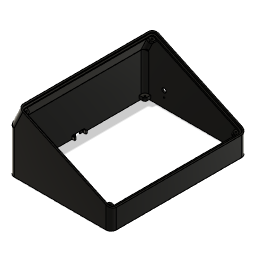
CP-BO Side v19 (Autodesk Fusion 360 design; units mm, degrees)
Autodesk Fusion 360 part; units mm, degrees
sketch "Esquisse1" plane through (0, 0, 0) normal (0, 0, 1) x (1, 0, 0)
  line L0 (17.7197, 122.5237) -> (198.9812, 38)
  line L1 (198.9812, 38) -> (0, 38) construction
  line L2 (198.9812, 38) -> (179.1229, -4.5863) construction
  line L3 (181.2616, 0) -> (-66.8807, 115.7106) construction
  line L4 (17.7197, 122.5237) -> (0, 84.5237)
  line L5 (0, 84.5237) -> (0, 0)
  line L6 (198.9812, 38) -> (198.9812, 0)
  line L7 (2.6, 0) -> (2.6, 83.3113) construction
  line L8 (0, 0) -> (198.9812, 0)
  line L9 (80, 0) -> (80, 93.4819) construction
  line L10 (20.0761, 121.4248) -> (0, 78.3715) construction
  dimension "d7" = 25
  dimension "d8" = 200
  dimension "d13" = 46.188
  dimension "d15" = 2.6
  dimension "d17" = 38
  dimension "d20" = 83.1247
  dimension "d21" = 197.5823
  dimension "d188" = 80
  dimension "d189" = 2.6
  dimension "d190" = 41.9284
  constraint perpendicular L0 L2
  constraint coincident L2 L3.start
  constraint parallel L0 L3
  constraint coincident L3 L4.end
  constraint perpendicular L3 L4
  constraint perpendicular L1 L6
  constraint coincident L3 L7.end
  constraint perpendicular L6 L8
  constraint coincident L3.start L8
  constraint perpendicular L5 L8
  constraint coincident L5.end L8.start
  constraint coincident L7.start L8
  constraint coincident L8 L9.start
  constraint perpendicular L8 L9
  constraint coincident L1.end L5
  constraint coincident L0 L9.end
  constraint vertical L9
  constraint coincident L0 L10.start
  constraint coincident L5 L10.end
  constraint parallel L4 L10
  measures "d7" angle of L0 L1
  measures "d8" distance of L0.start L0.end
  measures "d15" distance of L5 L7
  measures "d17" distance of L6.end L0.end
  measures "d188" distance of L5 L9
  measures "d189" distance of L4 L10
  measures "d190" distance of L3 L10.start
extrude "Largeur boitier" add sketch "Esquisse1" along normal blind 265 makes body 1
fillet "Congés boitier" radius 10 6 edges at (198.9812, 19, 0) (198.9812, 19, 265) (0, 42.2618, 265) (8.8598, 103.5237, 265) (8.8598, 103.5237, 0) (0, 42.2618, 0) on bodies 1
fillet "Congé arrière" radius 10 3 edges at (2.9289, 83.8743, 2.9289) (0, 84.5237, 132.5) (2.9289, 83.8743, 262.0711) on bodies 1
sketch "Esquisse6" plane through (50.0941, 107.4272, 0) normal (0.422618, 0.906308, 0) x (0, 0, -1)
  arc A0 (0, 25.7212) -> (-10, 35.7212) centre (-10, 25.7212) ccw
  line L0 (-10, 35.7212) -> (-255, 35.7212)
  arc A1 (-255, 35.7212) -> (-265, 25.7212) centre (-255, 25.7212) ccw
  line L1 (-265, 25.7212) -> (-265, -153.245)
  ellipse E0 centre (-255, -153.245) end of major axis (-255, -164.2788) minor radius 10 (-265, -153.245) -> (-255, -164.2788) ccw
  line L2 (-255, -164.2788) -> (-10, -164.2788)
  ellipse E1 centre (-10, -153.245) end of major axis (-10, -164.2788) minor radius 10 (-10, -164.2788) -> (0, -153.245) ccw
  line L3 (0, -153.245) -> (0, 25.7212)
  line L4 (-262.4, 25.7212) -> (-262.4, -153.245)
  spline S0 degree 3 poles (-262.4, -153.245) (-262.4, -155.3628) (-261.6582, -157.4606) (-260.4214, -158.9788) (-259.0049, -160.7177) (-256.9935, -161.6788) (-255, -161.6788) knots -1.570796 -1.570796 -1.570796 -1.570796 -0.838623 -0.838623 -0.838623 0 0 0 0
  line L5 (-255, -161.6788) -> (-10, -161.6788)
  spline S1 degree 3 poles (-10, -161.6788) (-8.1331, -161.6788) (-6.2517, -160.8417) (-4.8554, -159.301) (-3.5538, -157.8648) (-2.7132, -155.8209) (-2.6111, -153.7066) (-2.6037, -153.5529) (-2.6, -153.3989) (-2.6, -153.245) knots 0 0 0 0 0.785398 0.785398 0.785398 1.517572 1.517572 1.517572 1.570796 1.570796 1.570796 1.570796
  line L6 (-2.6, -153.245) -> (-2.6, 25.7212)
  arc A2 (-2.6, 25.7212) -> (-10, 33.1212) centre (-10, 25.7212) ccw
  line L7 (-10, 33.1212) -> (-255, 33.1212)
  arc A3 (-255, 33.1212) -> (-262.4, 25.7212) centre (-255, 25.7212) ccw
  dimension "d61" = -2.6
extrude "Trou supérieur (1)" cut sketch "Esquisse6" against normal blind 41.928 contours L4 S0 L5 S1 L6 A2 L7 A3 bodies 1
sketch "Esquisse7" plane through (0, 0, 0) normal (0, -1, 0) x (1, 0, 0)
  arc A0 (0, 10) -> (10, 0) centre (10, 10) ccw
  line L0 (10, 0) -> (188.9812, 0)
  arc A1 (188.9812, 0) -> (198.9812, 10) centre (188.9812, 10) ccw
  line L1 (198.9812, 10) -> (198.9812, 255)
  arc A2 (198.9812, 255) -> (188.9812, 265) centre (188.9812, 255) ccw
  line L2 (188.9812, 265) -> (10, 265)
  arc A3 (10, 265) -> (0, 255) centre (10, 255) ccw
  line L3 (0, 255) -> (0, 10)
  line L4 (2.6, 255) -> (2.6, 10)
  arc A4 (2.6, 10) -> (10, 2.6) centre (10, 10) ccw
  line L5 (10, 2.6) -> (188.9812, 2.6)
  arc A5 (188.9812, 2.6) -> (196.3812, 10) centre (188.9812, 10) ccw
  line L6 (196.3812, 10) -> (196.3812, 255)
  arc A6 (196.3812, 255) -> (188.9812, 262.4) centre (188.9812, 255) ccw
  line L7 (188.9812, 262.4) -> (10, 262.4)
  arc A7 (10, 262.4) -> (2.6, 255) centre (10, 255) ccw
  dimension "d64" = -2.6
extrude "Trou inférieur (2)" cut sketch "Esquisse7" against normal blind 83.311 contours L4 A4 L5 A5 L6 A6 L7 A7 bodies 1
sketch "Esquisse8" plane through (50.0941, 107.4272, 0) normal (0.422618, 0.906308, 0) x (0, 0, -1)
  line L0 (-262.4, -153.245) -> (-262.4, 25.7212)
  arc A0 (-255, 33.1212) -> (-262.4, 25.7212) centre (-255, 25.7212) ccw
  line L1 (-255, 33.1212) -> (-10, 33.1212)
  arc A1 (-2.6, 25.7212) -> (-10, 33.1212) centre (-10, 25.7212) ccw
  line L2 (-2.6, 25.7212) -> (-2.6, -153.245)
  spline S0 degree 3 poles (-2.6, -153.245) (-2.6, -153.3989) (-2.6037, -153.5529) (-2.6111, -153.7066) (-2.7132, -155.8209) (-3.5538, -157.8648) (-4.8554, -159.301) (-6.2517, -160.8417) (-8.1331, -161.6788) (-10, -161.6788) knots -1.570796 -1.570796 -1.570796 -1.570796 -1.517572 -1.517572 -1.517572 -0.785398 -0.785398 -0.785398 0 0 0 0
  line L3 (-10, -161.6788) -> (-255, -161.6788)
  spline S1 degree 3 poles (-255, -161.6788) (-256.9935, -161.6788) (-259.0049, -160.7177) (-260.4214, -158.9788) (-261.6582, -157.4606) (-262.4, -155.3628) (-262.4, -153.245) knots 0 0 0 0 0.838623 0.838623 0.838623 1.570796 1.570796 1.570796 1.570796
  arc A2 (0, 25.7212) -> (-10, 35.7212) centre (-10, 25.7212) ccw
  line L4 (-10, 35.7212) -> (-255, 35.7212)
  arc A3 (-255, 35.7212) -> (-265, 25.7212) centre (-255, 25.7212) ccw
  line L5 (-265, 25.7212) -> (-265, -153.245)
  ellipse E0 centre (-255, -153.245) end of major axis (-255, -164.2788) minor radius 10 (-265, -153.245) -> (-255, -164.2788) ccw
  line L6 (-255, -164.2788) -> (-10, -164.2788)
  ellipse E1 centre (-10, -153.245) end of major axis (-10, -164.2788) minor radius 10 (-10, -164.2788) -> (0, -153.245) ccw
  line L7 (0, -153.245) -> (0, 25.7212)
  line L8 (-259.4, -153.245) -> (-259.4, 25.7212)
  arc A4 (-255, 30.1212) -> (-259.4, 25.7212) centre (-255, 25.7212) ccw
  line L9 (-255, 30.1212) -> (-10, 30.1212)
  arc A5 (-5.6, 25.7212) -> (-10, 30.1212) centre (-10, 25.7212) ccw
  line L10 (-5.6, 25.7212) -> (-5.6, -153.245)
  spline S2 degree 3 poles (-5.6, -153.245) (-5.6, -153.3507) (-5.6026, -153.4564) (-5.6076, -153.5619) (-5.6716, -154.8868) (-6.2136, -156.2424) (-6.9303, -157.1147) (-6.9791, -157.1741) (-7.0285, -157.2314) (-7.0783, -157.2864) (-7.9373, -158.2342) (-9.0298, -158.6788) (-10, -158.6788) knots -1.570796 -1.570796 -1.570796 -1.570796 -1.517572 -1.517572 -1.517572 -0.832072 -0.832072 -0.832072 -0.785398 -0.785398 -0.785398 0 0 0 0
  line L11 (-10, -158.6788) -> (-255, -158.6788)
  spline S3 degree 3 poles (-255, -158.6788) (-256.0293, -158.6788) (-257.2154, -158.1645) (-258.0955, -157.0841) (-258.7978, -156.2219) (-259.331, -154.8622) (-259.3932, -153.5326) (-259.3977, -153.4365) (-259.4, -153.3405) (-259.4, -153.245) knots 0 0 0 0 0.838623 0.838623 0.838623 1.521425 1.521425 1.521425 1.570796 1.570796 1.570796 1.570796
  point P0 (-10, 25.7212)
  point P1 (-255, 25.7212)
  point P2 (-10, 25.7212)
  point P3 (-255, 25.7212)
  point P4 (-10, 25.7212)
  point P5 (-255, 25.7212)
  constraint parallel L0 L8
  constraint concentric A0 A4
  constraint parallel L1 L9
  constraint concentric A1 A5
  constraint parallel L2 L10
  constraint parallel L3 L11
  constraint tangent L8 A4
  constraint tangent A4 L9
  constraint tangent L9 A5
  constraint tangent A5 L10
extrude "Extrude17" add sketch "Esquisse8" along normal blind -9.2 and the other way blind 3.2 contours L0 A0 L1 A1 L2 S0 L3 S1 bodies 1
chamfer "Chamfer3" distance 3 angle 45 8 edges at (18.9069, 111.819, 132.5) (20.0749, 111.2743, 258.1113) (103.9939, 72.1422, 259.4) (188.7528, 32.6185, 257.9244) (190.0178, 32.0286, 132.5) (188.7559, 32.6171, 7.0783) (103.9939, 72.1422, 5.6) (20.0749, 111.2743, 6.8887) on bodies 1
sketch "Sketch22" plane through (50.0941, 107.4272, 0) normal (0.422618, 0.906308, 0) x (0, 0, -1)
  line L0 (-262.4, -153.245) -> (-262.4, 25.7212)
  arc A0 (-255, 33.1212) -> (-262.4, 25.7212) centre (-255, 25.7212) ccw
  line L1 (-255, 33.1212) -> (-10, 33.1212)
  arc A1 (-2.6, 25.7212) -> (-10, 33.1212) centre (-10, 25.7212) ccw
  line L2 (-2.6, 25.7212) -> (-2.6, -153.245)
  spline S0 degree 3 poles (-2.6, -153.245) (-2.6, -153.3989) (-2.6037, -153.5529) (-2.6111, -153.7066) (-2.7132, -155.8209) (-3.5538, -157.8648) (-4.8554, -159.301) (-6.2517, -160.8417) (-8.1331, -161.6788) (-10, -161.6788) knots -1.570796 -1.570796 -1.570796 -1.570796 -1.517572 -1.517572 -1.517572 -0.785398 -0.785398 -0.785398 0 0 0 0
  line L3 (-10, -161.6788) -> (-255, -161.6788)
  spline S1 degree 3 poles (-255, -161.6788) (-256.9935, -161.6788) (-259.0049, -160.7177) (-260.4214, -158.9788) (-261.6582, -157.4606) (-262.4, -155.3628) (-262.4, -153.245) knots 0 0 0 0 0.838623 0.838623 0.838623 1.570796 1.570796 1.570796 1.570796
  arc A2 (0, 25.7212) -> (-10, 35.7212) centre (-10, 25.7212) ccw
  line L4 (-10, 35.7212) -> (-255, 35.7212)
  arc A3 (-255, 35.7212) -> (-265, 25.7212) centre (-255, 25.7212) ccw
  line L5 (-265, 25.7212) -> (-265, -153.245)
  ellipse E0 centre (-255, -153.245) end of major axis (-255, -164.2788) minor radius 10 (-265, -153.245) -> (-255, -164.2788) ccw
  line L6 (-255, -164.2788) -> (-10, -164.2788)
  ellipse E1 centre (-10, -153.245) end of major axis (-10, -164.2788) minor radius 10 (-10, -164.2788) -> (0, -153.245) ccw
  line L7 (0, -153.245) -> (0, 25.7212)
  line L8 (-265, 35.7212) -> (-251, 35.7212)
  line L9 (-251, 35.7212) -> (-251, 25.7212)
  line L10 (-255, 21.7212) -> (-265, 21.7212)
  line L11 (-265, 21.7212) -> (-265, 35.7212)
  arc A4 (-255, 21.7212) -> (-251, 25.7212) centre (-255, 25.7212) ccw
  circle A5 centre (-255, 25.7212) radius 1.5
  line L12 (0, 35.7212) -> (-14, 35.7212)
  line L13 (-14, 35.7212) -> (-14, 25.7212)
  line L14 (-10, 21.7212) -> (0, 21.7212)
  line L15 (0, 21.7212) -> (0, 35.7212)
  arc A6 (-14, 25.7212) -> (-10, 21.7212) centre (-10, 25.7212) ccw
  circle A7 centre (-10, 25.7212) radius 1.5
  line L16 (0, -150.2788) -> (-10, -150.2788)
  line L17 (-14, -154.2788) -> (-14, -164.2788)
  line L18 (-14, -164.2788) -> (0, -164.2788)
  line L19 (0, -164.2788) -> (0, -150.2788)
  arc A8 (-10, -150.2788) -> (-14, -154.2788) centre (-10, -154.2788) ccw
  circle A9 centre (-10, -154.2788) radius 1.5
  line L20 (-265, -150.2788) -> (-255, -150.2788)
  line L21 (-251, -154.2788) -> (-251, -164.2788)
  line L22 (-251, -164.2788) -> (-265, -164.2788)
  line L23 (-265, -164.2788) -> (-265, -150.2788)
  arc A10 (-251, -154.2788) -> (-255, -150.2788) centre (-255, -154.2788) ccw
  circle A11 centre (-255, -154.2788) radius 1.5
  point P0 (-10, 25.7212)
  point P1 (-255, 25.7212)
  point P2 (-10, 25.7212)
  point P3 (-255, 25.7212)
  point P4 (-10, 25.7212)
  point P5 (-255, 25.7212)
  dimension "d153" = 14
  dimension "d154" = 14
  dimension "d155" = 4
  dimension "d156" = 3
  dimension "d157" = 14
  dimension "d158" = 14
  dimension "d159" = 4
  dimension "d160" = 3
  dimension "d161" = 14
  dimension "d162" = 14
  dimension "d163" = 4
  dimension "d164" = 3
  dimension "d165" = 14
  dimension "d166" = 14
  dimension "d167" = 4
  dimension "d168" = 3
  constraint horizontal L8
  constraint vertical L9
  constraint horizontal L10
  constraint vertical L11
  constraint coincident L4 L8.end
  constraint coincident L5 L10.end
  constraint tangent L9 A4
  constraint tangent L10 A4
  constraint concentric A4 A5
  constraint horizontal L12
  constraint vertical L13
  constraint horizontal L14
  constraint vertical L15
  constraint coincident L4 L12.end
  constraint coincident L7 L14.end
  constraint tangent L13 A6
  constraint tangent L14 A6
  constraint concentric A6 A7
  constraint horizontal L16
  constraint vertical L17
  constraint horizontal L18
  constraint vertical L19
  constraint coincident L6 L17.end
  constraint coincident L7 L16.start
  constraint tangent L16 A8
  constraint tangent L17 A8
  constraint concentric A8 A9
  constraint horizontal L20
  constraint vertical L21
  constraint horizontal L22
  constraint vertical L23
  constraint coincident L6 L21.end
  constraint coincident L5 L20.start
  constraint tangent L20 A10
  constraint tangent L21 A10
  constraint concentric A10 A11
  measures "d153" distance of L9 L11
  measures "d154" distance of L8 L10
  measures "d155" radius of A4
  measures "d156" diameter of A5
  measures "d157" distance of L13 L15
  measures "d158" distance of L12 L14
  measures "d159" radius of A6
  measures "d160" diameter of A7
  measures "d161" distance of L17 L19
  measures "d162" distance of L16 L18
  measures "d163" radius of A8
  measures "d164" diameter of A9
  measures "d165" distance of L21 L23
  measures "d166" distance of L20 L22
  measures "d167" radius of A10
  measures "d168" diameter of A11
extrude "Extrude18" add sketch "Sketch22" along normal blind -12 and the other way blind 6 contours L0 L3 S1 L5 E0 L6 L20 L21 L22 L23 | L0 L3 S1 L20 L21 A10 | L0 A0 L1 L9 L10 A4 | L2 S0 L3 L16 L17 A8 | L2 S0 L3 L6 E1 L7 L16 L17 L18 L19 | L1 A1 L2 L13 L14 A6 bodies 1
extrude "Extrude19" add 1 faces at (197.4103, 38.7325, 91.6667) along direction (-0.422618, -0.906308, 0) blind 5 on bodies 1 bodies 1
extrude "Extrude20" add 1 faces at (192.1591, 36.6206, 93) along direction (0.906308, -0.422618, 0) blind 7 on bodies 1 bodies 1
extrude "Extrude21" add 1 faces at (192.2508, 32.0896, 93) along direction (0.939693, 0.34202, 0) blind 3 draft 10 on bodies 1 bodies 1
sketch "Sketch19" plane through (0, 0, 0) normal (0, -1, 0) x (1, 0, 0)
  line L0 (2.6, 10) -> (2.6, 255)
  arc A0 (10, 262.4) -> (2.6, 255) centre (10, 255) ccw
  line L1 (10, 262.4) -> (188.9812, 262.4)
  arc A1 (196.3812, 255) -> (188.9812, 262.4) centre (188.9812, 255) ccw
  line L2 (196.3812, 255) -> (196.3812, 10)
  arc A2 (188.9812, 2.6) -> (196.3812, 10) centre (188.9812, 10) ccw
  line L3 (188.9812, 2.6) -> (10, 2.6)
  arc A3 (2.6, 10) -> (10, 2.6) centre (10, 10) ccw
  arc A4 (0, 10) -> (10, 0) centre (10, 10) ccw
  line L4 (10, 0) -> (188.9812, 0)
  arc A5 (188.9812, 0) -> (198.9812, 10) centre (188.9812, 10) ccw
  line L5 (198.9812, 10) -> (198.9812, 255)
  arc A6 (198.9812, 255) -> (188.9812, 265) centre (188.9812, 255) ccw
  line L6 (188.9812, 265) -> (10, 265)
  arc A7 (10, 265) -> (0, 255) centre (10, 255) ccw
  line L7 (0, 255) -> (0, 10)
  line L8 (0, 0) -> (14, 0)
  line L9 (14, 0) -> (14, 10)
  line L10 (10, 14) -> (0, 14)
  line L11 (0, 14) -> (0, 0)
  arc A8 (14, 10) -> (10, 14) centre (10, 10) ccw
  circle A9 centre (10, 10) radius 1.5
  line L12 (0, 265) -> (14, 265)
  line L13 (14, 265) -> (14, 255)
  line L14 (10, 251) -> (0, 251)
  line L15 (0, 251) -> (0, 265)
  arc A10 (10, 251) -> (14, 255) centre (10, 255) ccw
  circle A11 centre (10, 255) radius 1.5
  line L16 (198.9812, 265) -> (184.9812, 265)
  line L17 (184.9812, 265) -> (184.9812, 255)
  line L18 (188.9812, 251) -> (198.9812, 251)
  line L19 (198.9812, 251) -> (198.9812, 265)
  line L20 (198.9812, 14) -> (188.9812, 14)
  line L21 (184.9812, 10) -> (184.9812, 0)
  line L22 (184.9812, 0) -> (198.9812, 0)
  line L23 (198.9812, 0) -> (198.9812, 14)
  arc A12 (188.9812, 14) -> (184.9812, 10) centre (188.9812, 10) ccw
  circle A13 centre (188.9812, 10) radius 1.5
  arc A14 (184.9812, 255) -> (188.9812, 251) centre (188.9812, 255) ccw
  circle A15 centre (188.9812, 255) radius 1.5
  line L24 (0, 132.5) -> (2.6, 132.5) construction
  line L25 (0, 136.8) -> (1.3, 136.8)
  line L26 (1.3, 136.8) -> (1.3, 128.2)
  line L27 (1.3, 128.2) -> (0, 128.2)
  line L28 (0, 128.2) -> (0, 136.8)
  line L29 (2.6, 142.3) -> (1.3, 142.3)
  line L30 (1.3, 142.3) -> (1.3, 122.7)
  line L31 (1.3, 122.7) -> (2.6, 122.7)
  line L32 (2.6, 122.7) -> (2.6, 142.3)
  dimension "d112" = 14
  dimension "d113" = 14
  dimension "d114" = 4
  dimension "d115" = 3
  dimension "d116" = 14
  dimension "d117" = 14
  dimension "d118" = 4
  dimension "d119" = 3
  dimension "d120" = 14
  dimension "d121" = 14
  dimension "d122" = 14
  dimension "d123" = 14
  dimension "d124" = 4
  dimension "d125" = 3
  dimension "d126" = 4
  dimension "d127" = 3
  dimension "d137" = 1.3
  dimension "d138" = 19.6
  dimension "d139" = 8.6
  constraint horizontal L8
  constraint vertical L9
  constraint horizontal L10
  constraint vertical L11
  constraint tangent L9 A8
  constraint tangent L10 A8
  constraint concentric A3 A9
  constraint horizontal L12
  constraint vertical L13
  constraint horizontal L14
  constraint vertical L15
  constraint tangent L13 A10
  constraint tangent L14 A10
  constraint concentric A0 A11
  constraint horizontal L16
  constraint vertical L17
  constraint horizontal L18
  constraint vertical L19
  constraint coincident L6 L16.end
  constraint coincident L5 L18.end
  constraint coincident L6 L12.end
  constraint coincident L7 L14.end
  constraint coincident L4 L8.end
  constraint coincident L7 L10.end
  constraint horizontal L20
  constraint vertical L21
  constraint horizontal L22
  constraint vertical L23
  constraint coincident L4 L21.end
  constraint coincident L5 L20.start
  constraint tangent L20 A12
  constraint tangent L21 A12
  constraint concentric A12 A13
  constraint tangent L17 A14
  constraint tangent L18 A14
  constraint concentric A14 A15
  constraint midpoint L7 L24.start
  constraint midpoint L0 L24.end
  constraint horizontal L25
  constraint vertical L26
  constraint horizontal L27
  constraint vertical L28
  constraint coincident L7 L25.start
  constraint horizontal L29
  constraint vertical L30
  constraint horizontal L31
  constraint vertical L32
  constraint coincident L26 L30.end
  constraint coincident L0 L29.start
  constraint symmetric L24 L29 L31
  constraint symmetric L24 L25 L27
  measures "d112" distance of L8.start L8.end
  measures "d113" distance of L8.start L10.end
  measures "d114" radius of A8
  measures "d115" diameter of A9
  measures "d116" distance of L12.start L12.end
  measures "d117" distance of L12.start L14.end
  measures "d118" radius of A10
  measures "d119" diameter of A11
  measures "d120" distance of L16.start L16.end
  measures "d121" distance of L16.start L18.end
  measures "d122" distance of L20 L22
  measures "d123" distance of L21 L23
  measures "d124" radius of A12
  measures "d125" diameter of A13
  measures "d126" radius of A14
  measures "d127" diameter of A15
  measures "d137" distance of L30 L32
  measures "d138" distance of L29 L31
  measures "d139" distance of L25 L27
extrude "Support vis inférieures (1)" add sketch "Sketch19" along normal blind -9 and the other way blind 3 contours L0 L3 A3 L9 L10 A8 | L0 L3 A3 A4 L4 L7 L8 L9 L10 L11 | L0 A0 L1 L6 A7 L7 L12 L13 L14 L15 | L0 A0 L1 L13 L14 A10 | L2 A2 L3 L20 L21 A12 | L2 A2 L3 L4 A5 L5 L20 L21 L22 L23 | L1 A1 L2 L5 A6 L6 L16 L17 L18 L19 | L1 A1 L2 L17 L18 A14 bodies 1
extrude "trou micro-usb & Arduino" cut sketch "Sketch19" against normal blind 6 contours L0 L26 L29 L30 L31 L32 | L7 L25 L26 L27 L28 L30 bodies 1
sketch "Guide Arduino" plane through (2.6, 0, 0) normal (1, 0, 0) x (0, 0, -1)
  line L0 (-122.7, 6) -> (-122.7, 0)
  line L1 (-122.7, 0) -> (-10, 0)
  line L2 (-10, 0) -> (-10, 3)
  line L3 (-10, 3) -> (-14, 3)
  line L4 (-14, 3) -> (-14, 9)
  line L5 (-14, 9) -> (-10, 9)
  line L6 (-10, 9) -> (-10, 83.311)
  line L7 (-10, 83.311) -> (-255, 83.311)
  line L8 (-255, 83.311) -> (-255, 9)
  line L9 (-255, 9) -> (-251, 9)
  line L10 (-251, 9) -> (-251, 3)
  line L11 (-251, 3) -> (-255, 3)
  line L12 (-255, 3) -> (-255, 0)
  line L13 (-255, 0) -> (-142.3, 0)
  line L14 (-142.3, 0) -> (-142.3, 6)
  line L15 (-142.3, 6) -> (-122.7, 6)
  line L16 (-142.3, 0) -> (-144.8, 0)
  line L17 (-144.8, 0) -> (-144.8, 6)
  line L18 (-144.8, 6) -> (-142.3, 6)
  line L19 (-142.3, 6) -> (-142.3, 0)
  line L20 (-122.7, 0) -> (-120.2, 0)
  line L21 (-120.2, 0) -> (-120.2, 6)
  line L22 (-120.2, 6) -> (-122.7, 6)
  line L23 (-122.7, 6) -> (-122.7, 0)
  dimension "d142" = 2.5
  dimension "d143" = 2.5
  constraint horizontal L16
  constraint vertical L17
  constraint horizontal L18
  constraint vertical L19
  constraint coincident L13.end L14.start
  constraint horizontal L20
  constraint vertical L21
  constraint horizontal L22
  constraint vertical L23
  constraint coincident L0.end L1.start
  measures "d142" distance of L13.end L16.end
  measures "d143" distance of L0.end L20.end
extrude "Guide Arduino (1)" add sketch "Guide Arduino" along normal blind 5 separate body contours L0 L1 L20 L21 L22 L23 | L13 L14 L16 L17 L18 L19 makes body 2 at (4.2667, 2, 120.2) makes body 3 at (4.2667, 2, 144.8)
fillet "Guide Arduino (2)" radius 1 2 edges at (5.1, 6, 120.2) (5.1, 6, 144.8) on bodies 2 3
sketch "Esquisse23" plane through (0, 0, 2.6) normal (0, 0, 1) x (1, 0, 0)
  line L0 (10, 9) -> (14, 9)
  line L1 (14, 9) -> (14, 3)
  line L2 (14, 3) -> (10, 3)
  line L3 (10, 3) -> (10, 0)
  line L4 (10, 0) -> (188.9812, 0)
  line L5 (188.9812, 0) -> (188.9812, 3)
  line L6 (188.9812, 3) -> (184.9812, 3)
  line L7 (184.9812, 3) -> (184.9812, 9)
  line L8 (184.9812, 9) -> (188.9812, 9)
  line L9 (188.9812, 9) -> (188.9812, 29.4225)
  line L10 (188.9812, 29.4225) -> (181.2215, 33.041)
  line L11 (181.2215, 33.041) -> (182.4049, 35.5786)
  line L12 (182.4049, 35.5786) -> (26.5199, 108.269)
  line L13 (26.5199, 108.269) -> (25.3366, 105.7313)
  line L14 (25.3366, 105.7313) -> (21.7113, 107.4218)
  line L15 (21.7113, 107.4218) -> (10.4683, 83.311)
  line L16 (10.4683, 83.311) -> (10, 83.311)
  line L17 (9.0632, 80.2978) -> (10, 79.861)
  line L18 (10, 79.861) -> (10, 9)
  circle A0 centre (40, 30) radius 4.2
  line L19 (40, 65) -> (40, 0) construction
  circle A1 centre (40, 18) radius 1.3
  line L20 (10, 83.311) -> (10, 82.3067)
  line L21 (10, 82.3067) -> (9.0632, 80.2978)
  dimension "d179" = 8.4
  dimension "d180" = 30
  dimension "d181" = 30
  dimension "d182" = 2.6
  dimension "d183" = 12
  constraint coincident L4 L19.end
  constraint perpendicular L4 L19
  constraint coincident A0.centre L19
  constraint coincident L19 A1.centre
  measures "d179" diameter of A0
  measures "d180" distance of L18 A0.centre
  measures "d181" distance of L4 A0.centre
  measures "d182" diameter of A1
  measures "d183" distance of A0.centre A1.centre
extrude "Extrusion22" cut sketch "Esquisse23" against normal blind 3 contours A0 bodies 1
extrude "Extrusion23" cut sketch "Esquisse23" against normal blind 2 contours A1 bodies 1
